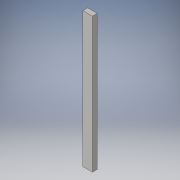
# Autodesk Inventor part: Cabinet Support Frame Center Vertical Bar
Saved by Autodesk Inventor 2016 (Build 200138000, 138)
## iProperties
Created: 2018-02-03
Part Number: Cabinet Support Frame Center Vertical Bar
Material: Generic
Document SubType Name: Modeling
Designer: dash
Density: 1 g/cm^3
Appearance: Default
Author: dash
Autodesk Inventor part; units mm, degrees
ref_plane "YZ Plane" through (0, 0, 0) normal (1, 0, 0) x (0, 1, 0)
ref_plane "XZ Plane" through (0, 0, 0) normal (0, 1, 0) x (-1, 0, 0)
ref_plane "XY Plane" through (0, 0, 0) normal (0, 0, 1) x (1, 0, 0)
sketch "Sketch1" plane through (0, 0, 0) normal (0, 0, 1) x (1, 0, 0)
  line L0 (657.7721, 618.925) -> (695.8721, 618.925)
  line L1 (695.8721, 618.925) -> (695.8721, 82.35)
  line L2 (695.8721, 82.35) -> (657.7721, 82.35)
  line L3 (657.7721, 82.35) -> (657.7721, 618.925)
  point P0 (0, 0)
  dimension "d0" = 536.575
  dimension "d1" = 38.1
  constraints: 8 end point, 2 parallel, 1 horizontal, 1 perpendicular
  measures "d0" distance of L0.end L1.end
  measures "d1" distance of L1.end L2.end
extrude "Extrusion1" add sketch "Sketch1" along normal blind 19.05
body "Solid1"
